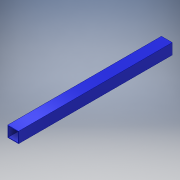
# Autodesk Inventor part: bluethingfortable
Saved by Autodesk Inventor 2017 (Build 210142000, 142)
## iProperties
Created: 2018-08-24
Part Number: bluethingfortable
Material: Generic
Document SubType Name: Modeling
Designer: emmacarlisle
Density: 1 g/cm^3
Appearance: Blue - Wall Paint - Glossy
Author: emmacarlisle
Autodesk Inventor part; units mm, degrees
ref_plane "YZ Plane" through (0, 0, 0) normal (1, 0, 0) x (0, 1, 0)
ref_plane "XZ Plane" through (0, 0, 0) normal (0, 1, 0) x (-1, 0, 0)
ref_plane "XY Plane" through (0, 0, 0) normal (0, 0, 1) x (1, 0, 0)
sketch "Sketch1" plane through (0, 0, 0) normal (0, 0, 1) x (1, 0, 0)
  line L0 (5.3443, -30.8421) -> (105.3443, -30.8421)
  line L1 (105.3443, -30.8421) -> (105.3443, 69.1579)
  line L2 (105.3443, 69.1579) -> (5.3443, 69.1579)
  line L3 (5.3443, 69.1579) -> (5.3443, -30.8421)
  line L4 (10.3443, 64.1579) -> (100.3443, 64.1579)
  line L5 (100.3443, 64.1579) -> (100.3443, -25.8421)
  line L6 (100.3443, -25.8421) -> (10.3443, -25.8421)
  line L7 (10.3443, -25.8421) -> (10.3443, 64.1579)
  point P0 (0, 0)
  dimension "d0" = 100
  dimension "d1" = 100
  dimension "d2" = 5
  dimension "d3" = 5
  dimension "d4" = 5
  dimension "d5" = 5
  constraints: 16 end point, 4 parallel, 2 horizontal, 2 perpendicular
  measures "d0" distance of L2.end L1.end
  measures "d1" distance of L2.end L0.start
  measures "d2" distance between parallel lines of L7 L3
  measures "d3" distance between parallel lines of L2 L4
  measures "d4" distance between parallel lines of L1 L5
  measures "d5" distance between parallel lines of L0 L6
extrude "Extrusion1" add sketch "Sketch1" along normal blind 1420
body "Solid1"
